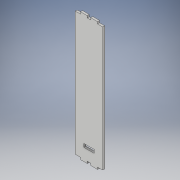
# Autodesk Inventor part: 4 binnen dikke cover plaat
Saved by Autodesk Inventor 2019 (Build 230136000, 136)
## iProperties
Created: 2021-01-22
Part Number: 4 binnen dikke cover plaat
Material: Generic
Document SubType Name: Sheet Metal
Designer: Stefan
Density: 1 g/cm^3
Sheet Metal Rule: Default_mm
Appearance: Default
Author: Stefan
Autodesk Inventor part; units mm, degrees
ref_plane "YZ Plane" through (0, 0, 0) normal (1, 0, 0) x (0, 1, 0)
ref_plane "XZ Plane" through (0, 0, 0) normal (0, 1, 0) x (-1, 0, 0)
ref_plane "XY Plane" through (0, 0, 0) normal (0, 0, 1) x (1, 0, 0)
sketch "Sketch1" plane through (0, 0, 0) normal (0, 0, 1) x (1, 0, 0)
  line L0 (20, -90.5) -> (20, 90.5)
  line L1 (-20, 90.5) -> (-20, -90.5)
  line L2 (-20, -90.5) -> (20, 90.5) construction
  line L3 (20, -90.5) -> (-20, 90.5) construction
  line L4 (-2.5, 90.5) -> (-2.5, 93.5)
  line L5 (-2.5, 93.5) -> (-12.5, 93.5)
  line L6 (-12.5, 93.5) -> (-12.5, 90.5)
  line L7 (12.5, 90.5) -> (12.5, 93.5)
  line L8 (12.5, 93.5) -> (2.5, 93.5)
  line L9 (2.5, 93.5) -> (2.5, 90.5)
  line L10 (12.5, 90.5) -> (20, 90.5)
  line L11 (-2.5, 90.5) -> (2.5, 90.5)
  line L12 (-20, 90.5) -> (-12.5, 90.5)
  line L13 (-20, -90.5) -> (-12.5, -90.5)
  line L14 (-12.5, -90.5) -> (-12.5, -93.5)
  line L15 (-12.5, -93.5) -> (-2.5, -93.5)
  line L16 (-2.5, -93.5) -> (-2.5, -90.5)
  line L17 (-2.5, -90.5) -> (2.5, -90.5)
  line L18 (2.5, -90.5) -> (2.5, -93.5)
  line L19 (2.5, -93.5) -> (12.5, -93.5)
  line L20 (12.5, -93.5) -> (12.5, -90.5)
  line L21 (12.5, -90.5) -> (20, -90.5)
  point P0 (0, 0)
  dimension "d0" = 40
  dimension "d1" = 181
  dimension "d2" = 10
  dimension "d3" = 3
  dimension "d4" = 7.5
  dimension "d5" = 10
  dimension "d6" = 3
  dimension "d7" = 5
  dimension "d8" = 7.5
  dimension "d9" = 3
  dimension "d10" = 10
  dimension "d11" = 5
  dimension "d12" = 3
  dimension "d13" = 10
  dimension "d14" = 3
  dimension "d15" = 12.462
  dimension "d16" = 90
  dimension "d17" = 0
  constraints: 44 end point, 6 parallel, 5 point on line, 4 perpendicular, 2 collinear, 2 horizontal, 2 midpoint
  measures "d0" distance of L1.start L0.end
  measures "d1" distance of L0.end L0.start
  measures "d2" distance of L5.end L4.end
  measures "d3" distance of L4.end L4.start
  measures "d4" distance between parallel lines of L6 L1
  measures "d5" distance of L8.end L7.end
  measures "d6" distance of L7.end L7.start
  measures "d7" distance between parallel lines of L9 L4
  measures "d8" distance of L1.end L13.end
  measures "d9" distance of L13.end L14.end
  measures "d10" distance of L14.end L15.end
  measures "d11" distance of L16.end L17.end
  measures "d12" distance of L17.end L18.end
  measures "d13" distance of L18.end L19.end
  measures "d14" distance of L19.end L20.end
  measures "d15" angle of L3 L0
  measures "d16" angle of L5 L0
  measures "d17" distance between parallel lines of L11 L10
extrude "Extrusion1" add sketch "Sketch1" along normal blind 3
sketch "Sketch2" plane through (0, 0, 3) normal (0, 0, 1) x (1, 0, 0)
  line L0 (-7.5, -70.5) -> (7.5, -70.5)
  line L1 (7.5, -70.5) -> (7.5, -75.5)
  line L2 (7.5, -75.5) -> (-7.5, -75.5)
  line L3 (-7.5, -75.5) -> (-7.5, -70.5)
  line L4 (-7.5, -70.5) -> (7.5, -75.5) construction
  line L5 (7.5, -70.5) -> (-7.5, -75.5) construction
  line L6 (-2.5, -90.5) -> (2.5, -90.5) projected
  line L7 (-20, 90.5) -> (-20, -90.5) projected
  point P0 (0, 0)
  point P1 (0, -73)
  dimension "d20" = 15
  dimension "d21" = 5
  dimension "d22" = 15
  dimension "d23" = 12.5
  constraints: 12 end point, 2 midpoint, 2 parallel, 1 horizontal, 1 perpendicular
  measures "d20" distance of L1.end L2.end
  measures "d21" distance of L0.end L1.end
  measures "d22" distance between parallel lines of L2 L6
  measures "d23" distance between parallel lines of L7 L3
extrude "Extrusion2" cut sketch "Sketch2" against normal blind 10
equation "\"BendRadius\" = Thickness"
equation "\"BendReliefWidth\" = Thickness"
equation "\"BendReliefDepth\" = 0.5 * Thickness"
equation "\"CornerReliefSize\" = 4 * Thickness"
equation "\"MinimumRemnant\" = 2 * Thickness"
equation "\"TransitionRadius\" = BendRadius"
equation "\"JacobiRadiusSize\" = BendRadius"
equation "\"GapSize\" = Thickness"
equation "\"Thickness\" = 0.5"
body "Solid1"
